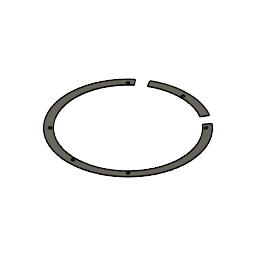
LED_Strip_Cover (Autodesk Fusion 360 design; units mm, degrees)
Autodesk Fusion 360 part; units mm, degrees
sketch "Sketch1" plane through (0, 0, 0) normal (0, 0, 1) x (1, 0, 0)
  circle A0 centre (0, 0) radius 102
  circle A1 centre (0, 0) radius 90
  circle A2 centre (0, 0) radius 94 construction
  circle A3 centre (-0.0983, 93.9999) radius 2
  circle A4 centre (-0.0084, -94) radius 2
  line L0 (0, 0) -> (66.468, 66.468) construction
  line L1 (0, 0) -> (94, 0) construction
  line L2 (-160, 0) -> (153.4074, 0) construction
  line L3 (0, 0) -> (-66.468, 66.468) construction
  line L4 (0, 0) -> (94, 0) construction
  circle A5 centre (-66.468, 66.468) radius 2
  circle A6 centre (66.468, 66.468) radius 2
  circle A7 centre (-66.468, -66.468) radius 2
  circle A8 centre (66.468, -66.468) radius 2
  dimension "d1" = 204
  dimension "d2" = 180
  dimension "d3" = 188
  dimension "d4" = 4
  dimension "d5" = 4
  dimension "d6" = 45
  dimension "d7" = 135
  dimension "d8" = 4
  dimension "d9" = 4
  constraint coincident A0.centre A1.centre
  constraint coincident A2 A3.centre
  constraint coincident A2 A4.centre
  constraint horizontal L1
  constraint parallel L1 L2
  constraint horizontal L4
  constraint coincident L3.end A5.centre
  constraint coincident L0.end A6.centre
  constraint symmetric L2 A5 A7
  constraint symmetric L2 A6 A8
  measures "d1" diameter of A0
  measures "d2" diameter of A1
  measures "d3" diameter of A2
  measures "d4" diameter of A3
  measures "d5" diameter of A4
  measures "d6" angle of L0 L1
  measures "d7" angle of L3 L4
  measures "d8" diameter of A5
  measures "d9" diameter of A6
extrude "Extrude1" add sketch "Sketch1" along normal blind 1 makes body 1
sketch "Sketch2" plane through (0, 0, 1) normal (0, 0, 1) x (-1, 0, 0)
  circle A0 centre (66.468, -66.468) radius 2
  circle A1 centre (0.0983, -93.9999) radius 2
  circle A2 centre (-66.468, 66.468) radius 2
  circle A3 centre (66.468, 66.468) radius 2
  circle A4 centre (0, 0) radius 90
  circle A5 centre (0.0084, 94) radius 2
  circle A6 centre (-66.468, -66.468) radius 2
  circle A7 centre (0, 0) radius 102
  line L0 (57.8509, -68.944) -> (65.5643, -78.1365)
  line L1 (0, 0) -> (102, 0) construction
  line L2 (45, -77.9423) -> (51, -88.3346)
  line L3 (0, 0) -> (102, 0) construction
  line L4 (-45, -77.9423) -> (-51, -88.3346)
  line L5 (0, 0) -> (102, 0) construction
  line L6 (-57.8509, -68.944) -> (-65.5643, -78.1365)
  line L7 (0, 0) -> (102, 0) construction
  dimension "d12" = 50
  dimension "d13" = 60
  dimension "d14" = 120
  dimension "d15" = 130
  constraint horizontal L1
  constraint coincident A4.centre A7.centre
  constraint horizontal L3
  constraint horizontal L5
  constraint horizontal L7
  constraint coincident A4 L0.start
  constraint coincident A4 L2.start
  constraint coincident A4 L4.start
  constraint coincident A4 L6.start
  measures "d12" angle of L0 L1
  measures "d13" angle of L2 L3
  measures "d14" angle of L4 L5
  measures "d15" angle of L6 L7
extrude "Extrude2" cut sketch "Sketch2" against normal blind 2 contours A4 A7 L4 L6 | A4 A7 L0 L2 bodies 1 makes body 2 at (-40.3818, 89.0208, 0)
extrude "Extrude3" cut 2 faces at (75.256, -58.3928, 1) (-40.3818, 89.0208, 1) along direction (0, 0, -1) blind 0.5 on bodies 1 2 bodies 1 2
